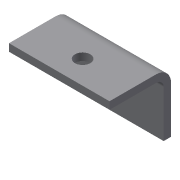
# Autodesk Inventor part: Chain Tension - L Bracket - Base
Saved by Autodesk Inventor 2015 (Build 190159000, 159)
## iProperties
Created: 2015-02-01
Part Number: Chain Tension - L Bracket - Base
Material: Generic
Document SubType Name: Sheet Metal
Designer: Tanner
Density: 1 g/cm^3
Sheet Metal Rule: Default
Appearance: Default
Author: Tanner
Autodesk Inventor part; units mm, degrees
ref_plane "YZ Plane" through (0, 0, 0) normal (1, 0, 0) x (0, 1, 0)
ref_plane "XZ Plane" through (0, 0, 0) normal (0, 1, 0) x (-1, 0, 0)
ref_plane "XY Plane" through (0, 0, 0) normal (0, 0, 1) x (1, 0, 0)
sketch "Sketch1" plane through (0, 0, 0) normal (0, 0, 1) x (1, 0, 0)
  line L0 (0, 0) -> (41.5036, 0)
  line L1 (41.5036, 0) -> (41.5036, 25.4)
  line L2 (41.5036, 25.4) -> (0, 25.4)
  line L3 (0, 25.4) -> (0, 0)
  dimension "d0" = 41.5036
  dimension "d1" = 25.4
  measures "d0" distance of L2.end L1.end
  measures "d1" distance of L1.end L0.end
extrude "Plate1" add sketch "Sketch1" along normal blind 3.048
sketch "Sketch3" plane through (0, 22.352, 0) normal (0, 1, 0) x (-1, 0, 0)
  line L0 (-41.5036, 0) -> (0, 0)
  line L1 (0, 0) -> (0, 25.4)
  line L2 (0, 25.4) -> (-41.5036, 25.4)
  line L3 (-41.5036, 25.4) -> (-41.5036, 0)
  constraints: 6 end point, 1 horizontal, 1 perpendicular, 1 vertical
edge flange "Flange2" height 25.4 angle 90 thickness 3.048 bend radius 3.048 thickness toward (0, 1, 0) relief tear relief width 3.048 relief depth 1.524 edges at (20.7518, 25.4, 3.048) wall of the first edge with corners at (41.5036, 22.352, 0) (0, 22.352, 0) (0, 22.352, 25.4) (41.5036, 22.352, 25.4)
bend "Bend2"
corner "Corner2"
hole "Hole1" at (20.7518, 22.352, 15.748) direction (0, 1, 0) diameter 6.35 end through all
equation "\"d30\" = Thickness"
equation "\"d13\" = BendReliefWidth"
equation "\"d14\" = BendReliefDepth"
equation "\"d15\" = MinimumRemnant"
equation "\"d16\" = BendRadius"
equation "\"d19\" = BendRadius"
equation "\"d20\" = CornerReliefSize"
equation "\"d21\" = GapSize"
equation "\"d22\" = JacobiRadiusSize"
equation "\"BendRadius\" = Thickness"
equation "\"BendReliefWidth\" = Thickness"
equation "\"BendReliefDepth\" = 0.5 * Thickness"
equation "\"CornerReliefSize\" = 4 * Thickness"
equation "\"MinimumRemnant\" = 2 * Thickness"
equation "\"TransitionRadius\" = BendRadius"
equation "\"JacobiRadiusSize\" = BendRadius"
equation "\"GapSize\" = Thickness"
equation "\"d2\" = BendRadius"
equation "\"Thickness\" = 3.048"
body "Solid1"
